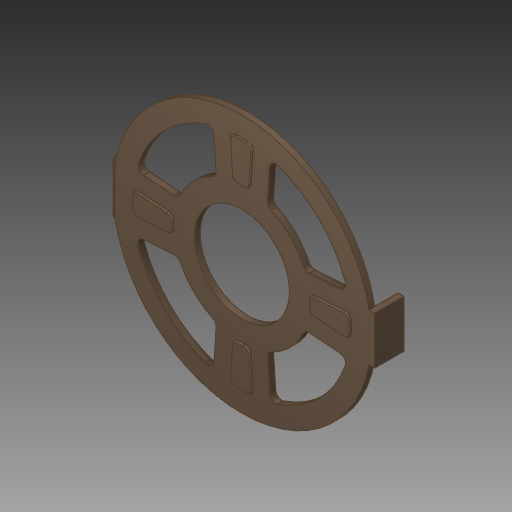
# Autodesk Inventor part: SŁONECZKO
Saved by Autodesk Inventor 2017 SP1 (Build 210196100, 196)
## iProperties
Created: 2021-01-06
Part Number: SŁONECZKO
Material: Stal
Document SubType Name: Modeling
Designer: Napoleon
Mass: 0.893655 g
Surface Area: 6.07713 cm^2
Volume: 0.113841 cm^3
Density: 7.85 g/cm^3
Appearance: Anodowany - brązowy
Author: Napoleon
Autodesk Inventor part; units mm, degrees
ref_plane "YZ Plane" through (0, 0, 0) normal (1, 0, 0) x (0, 1, 0)
ref_plane "XZ Plane" through (0, 0, 0) normal (0, 1, 0) x (-1, 0, 0)
ref_plane "XY Plane" through (0, 0, 0) normal (0, 0, 1) x (1, 0, 0)
sketch "Szkic1" plane through (0, 0, 0) normal (0, 0, 1) x (1, 0, 0)
  circle A0 centre (0, 0) radius 4.05
  line L0 (-11.3, 2.025) -> (-11.3, -2.025)
  line L1 (-10.8, 2.025) -> (-11.3, 2.025)
  line L2 (-9.2716, 0.9962) -> (-5.7517, 0.7466)
  line L3 (-9.0036, 2.4272) -> (-5.3787, 2.1701)
  line L4 (-9.2716, 0.9962) -> (-5.8, 0.75)
  line L5 (-9.2716, -0.9962) -> (-5.7517, -0.7466)
  line L6 (-9.0036, -2.4272) -> (-5.3787, -2.1701)
  line L7 (-9.2716, -0.9962) -> (-5.8, -0.75)
  line L8 (-2.4272, -9.0036) -> (-2.1701, -5.3787)
  line L9 (-0.9962, -9.2716) -> (-0.7466, -5.7517)
  line L10 (-0.9962, -9.2716) -> (-0.75, -5.8)
  line L11 (0.9962, -9.2716) -> (0.7466, -5.7517)
  line L12 (0.9962, -9.2716) -> (0.75, -5.8)
  line L13 (2.4272, -9.0036) -> (2.1701, -5.3787)
  line L14 (9.0036, -2.4272) -> (5.3787, -2.1701)
  line L15 (9.2716, -0.9962) -> (5.7517, -0.7466)
  line L16 (9.2716, -0.9962) -> (5.8, -0.75)
  line L17 (9.2716, 0.9962) -> (5.7517, 0.7466)
  line L18 (9.2716, 0.9962) -> (5.8, 0.75)
  line L19 (9.0036, 2.4272) -> (5.3787, 2.1701)
  line L20 (2.4272, 9.0036) -> (2.1701, 5.3787)
  line L21 (0.9962, 9.2716) -> (0.7466, 5.7517)
  line L22 (0.9962, 9.2716) -> (0.75, 5.8)
  line L23 (-0.9962, 9.2716) -> (-0.7466, 5.7517)
  line L24 (-0.9962, 9.2716) -> (-0.75, 5.8)
  line L25 (-2.4272, 9.0036) -> (-2.1701, 5.3787)
  arc A1 (0.9962, 9.2716) -> (-0.9962, 9.2716) centre (0, 0) ccw
  arc A2 (0.7466, 5.7517) -> (-0.7466, 5.7517) centre (0, 0) ccw
  arc A3 (5.3787, 2.1701) -> (2.1701, 5.3787) centre (0, 0) ccw
  arc A4 (9.0036, 2.4272) -> (2.4272, 9.0036) centre (0, 0) ccw
  arc A5 (9.2716, -0.9962) -> (9.2716, 0.9962) centre (0, 0) ccw
  arc A6 (5.7517, -0.7466) -> (5.7517, 0.7466) centre (0, 0) ccw
  arc A7 (2.4272, -9.0036) -> (9.0036, -2.4272) centre (0, 0) ccw
  arc A8 (2.1701, -5.3787) -> (5.3787, -2.1701) centre (0, 0) ccw
  arc A9 (-0.7466, -5.7517) -> (0.7466, -5.7517) centre (0, 0) ccw
  arc A10 (-0.9962, -9.2716) -> (0.9962, -9.2716) centre (0, 0) ccw
  arc A11 (-9.0036, -2.4272) -> (-2.4272, -9.0036) centre (0, 0) ccw
  arc A12 (-5.3787, -2.1701) -> (-2.1701, -5.3787) centre (0, 0) ccw
  arc A13 (-2.1701, 5.3787) -> (-5.3787, 2.1701) centre (0, 0) ccw
  arc A14 (-5.7517, 0.7466) -> (-5.7517, -0.7466) centre (0, 0) ccw
  arc A15 (-2.4272, 9.0036) -> (-9.0036, 2.4272) centre (0, 0) ccw
  arc A16 (-9.2716, 0.9962) -> (-9.2716, -0.9962) centre (0, 0) ccw
  line L26 (-10.8, -2.025) -> (-11.3, -2.025)
  arc A17 (-10.7083, -2.5164) -> (-2.5164, -10.7083) centre (0, 0) ccw
  arc A18 (-10.812, -2.025) -> (10.812, -2.025) centre (0, 0) ccw
  arc A19 (-2.5164, 10.7083) -> (-10.7083, 2.5164) centre (0, 0) ccw
  arc A20 (10.812, 2.025) -> (-10.812, 2.025) centre (0, 0) ccw
  line L27 (11.3, 2.025) -> (11.3, -2.025)
  line L28 (10.8, 2.025) -> (11.3, 2.025)
  line L29 (10.8, -2.025) -> (11.3, -2.025)
  dimension "d19" = 360
  constraints: 60 end point, 42 point on circle, 21 centre point, 4 point on line, 3 coincident, 65 other
extrude "Wyciągnięcie proste1" add sketch "Szkic1" against normal blind 0.5
fillet "Zaokrąglenie1" radius 0.5 32 edges at (-9.2716, 0.9962, -0.25) (-5.7517, 0.7466, -0.25) (-5.7517, -0.7466, -0.25) (-9.2716, -0.9962, -0.25) (-9.0036, 2.4272, -0.25) (-5.3787, 2.1701, -0.25) (-2.1701, 5.3787, -0.25) (-2.4272, 9.0036, -0.25) (-0.9962, 9.2716, -0.25) (-0.7466, 5.7517, -0.25) (0.7466, 5.7517, -0.25) (0.9962, 9.2716, -0.25) (2.4272, 9.0036, -0.25) (2.1701, 5.3787, -0.25) (5.3787, 2.1701, -0.25) (9.0036, 2.4272, -0.25) (5.7517, 0.7466, -0.25) (5.7517, -0.7466, -0.25) (9.2716, -0.9962, -0.25) (9.2716, 0.9962, -0.25) (5.3787, -2.1701, -0.25) (9.0036, -2.4272, -0.25) (2.1701, -5.3787, -0.25) (2.4272, -9.0036, -0.25) (-0.7466, -5.7517, -0.25) (0.7466, -5.7517, -0.25) (0.9962, -9.2716, -0.25) (-0.9962, -9.2716, -0.25) (-2.1701, -5.3787, -0.25) (-2.4272, -9.0036, -0.25) (-9.0036, -2.4272, -0.25) (-5.3787, -2.1701, -0.25)
sketch "Szkic2" plane through (0, 0, -0.5) normal (0, 0, -1) x (-1, 0, 0)
  line L0 (-11.3, 2.025) -> (-10.8, 2.025)
  line L1 (-11.3, 2.025) -> (-10.8, 2.025)
  line L2 (-10.8, 2.025) -> (-10.8, -2.025)
  line L3 (-10.8, -2.025) -> (-11.3, -2.025)
  line L4 (-11.3, -2.025) -> (-11.3, 2.025)
  line L5 (11.3, 2.025) -> (10.8, 2.025)
  line L6 (10.8, 2.025) -> (10.8, -2.025)
  line L7 (10.8, -2.025) -> (11.3, -2.025)
  line L8 (11.3, -2.025) -> (11.3, 2.025)
  circle A0 centre (0, 0) radius 4.05 projected
  arc A1 (-3.0447, 8.8139) -> (-8.8139, 3.0447) centre (0, 0) ccw projected
  arc A2 (-2.3827, 8.3767) -> (-3.0447, 8.8139) centre (-2.8815, 8.3413) ccw projected
  line L9 (-2.3827, 8.3767) -> (-2.1951, 5.7304) projected
  arc A3 (-2.48, 5.243) -> (-2.1951, 5.7304) centre (-2.6938, 5.695) ccw projected
  arc A4 (-2.48, 5.243) -> (-5.243, 2.48) centre (0, 0) ccw projected
  arc A5 (-5.7304, 2.1951) -> (-5.243, 2.48) centre (-5.695, 2.6938) ccw projected
  line L10 (-5.7304, 2.1951) -> (-8.3767, 2.3827) projected
  arc A6 (-8.8139, 3.0447) -> (-8.3767, 2.3827) centre (-8.3413, 2.8815) ccw projected
  arc A7 (-8.8139, -3.0447) -> (-3.0447, -8.8139) centre (0, 0) ccw projected
  arc A8 (-8.3767, -2.3827) -> (-8.8139, -3.0447) centre (-8.3413, -2.8815) ccw projected
  line L11 (-8.3767, -2.3827) -> (-5.7304, -2.1951) projected
  arc A9 (-5.243, -2.48) -> (-5.7304, -2.1951) centre (-5.695, -2.6938) ccw projected
  arc A10 (-5.243, -2.48) -> (-2.48, -5.243) centre (0, 0) ccw projected
  arc A11 (-2.1951, -5.7304) -> (-2.48, -5.243) centre (-2.6938, -5.695) ccw projected
  line L12 (-2.1951, -5.7304) -> (-2.3827, -8.3767) projected
  arc A12 (-3.0447, -8.8139) -> (-2.3827, -8.3767) centre (-2.8815, -8.3413) ccw projected
  arc A13 (3.0447, -8.8139) -> (8.8139, -3.0447) centre (0, 0) ccw projected
  arc A14 (2.3827, -8.3767) -> (3.0447, -8.8139) centre (2.8815, -8.3413) ccw projected
  line L13 (2.3827, -8.3767) -> (2.1951, -5.7304) projected
  arc A15 (2.48, -5.243) -> (2.1951, -5.7304) centre (2.6938, -5.695) ccw projected
  arc A16 (2.48, -5.243) -> (5.243, -2.48) centre (0, 0) ccw projected
  arc A17 (5.7304, -2.1951) -> (5.243, -2.48) centre (5.695, -2.6938) ccw projected
  line L14 (5.7304, -2.1951) -> (8.3767, -2.3827) projected
  arc A18 (8.8139, -3.0447) -> (8.3767, -2.3827) centre (8.3413, -2.8815) ccw projected
  arc A19 (5.243, 2.48) -> (2.48, 5.243) centre (0, 0) ccw projected
  arc A20 (2.1951, 5.7304) -> (2.48, 5.243) centre (2.6938, 5.695) ccw projected
  line L15 (2.1951, 5.7304) -> (2.3827, 8.3767) projected
  arc A21 (3.0447, 8.8139) -> (2.3827, 8.3767) centre (2.8815, 8.3413) ccw projected
  arc A22 (8.8139, 3.0447) -> (3.0447, 8.8139) centre (0, 0) ccw projected
  arc A23 (8.3767, 2.3827) -> (8.8139, 3.0447) centre (8.3413, 2.8815) ccw projected
  line L16 (8.3767, 2.3827) -> (5.7304, 2.1951) projected
  arc A24 (5.243, 2.48) -> (5.7304, 2.1951) centre (5.695, 2.6938) ccw projected
  arc A25 (0.4886, 9.3122) -> (-0.4886, 9.3122) centre (0, 0) ccw projected
  arc A26 (0.9612, 8.7775) -> (0.4886, 9.3122) centre (0.4624, 8.8129) ccw projected
  line L17 (0.9612, 8.7775) -> (0.7825, 6.2582) projected
  arc A27 (0.2612, 5.7941) -> (0.7825, 6.2582) centre (0.2838, 6.2936) ccw projected
  arc A28 (0.2612, 5.7941) -> (-0.2612, 5.7941) centre (0, 0) ccw projected
  arc A29 (-0.7825, 6.2582) -> (-0.2612, 5.7941) centre (-0.2838, 6.2936) ccw projected
  line L18 (-0.7825, 6.2582) -> (-0.9612, 8.7775) projected
  arc A30 (-0.4886, 9.3122) -> (-0.9612, 8.7775) centre (-0.4624, 8.8129) ccw projected
  arc A31 (-9.3122, 0.4886) -> (-9.3122, -0.4886) centre (0, 0) ccw projected
  arc A32 (-8.7775, 0.9612) -> (-9.3122, 0.4886) centre (-8.8129, 0.4624) ccw projected
  line L19 (-8.7775, 0.9612) -> (-6.2582, 0.7825) projected
  arc A33 (-5.7941, 0.2612) -> (-6.2582, 0.7825) centre (-6.2936, 0.2838) ccw projected
  arc A34 (-5.7941, 0.2612) -> (-5.7941, -0.2612) centre (0, 0) ccw projected
  arc A35 (-6.2582, -0.7825) -> (-5.7941, -0.2612) centre (-6.2936, -0.2838) ccw projected
  line L20 (-6.2582, -0.7825) -> (-8.7775, -0.9612) projected
  arc A36 (-9.3122, -0.4886) -> (-8.7775, -0.9612) centre (-8.8129, -0.4624) ccw projected
  arc A37 (-0.4886, -9.3122) -> (0.4886, -9.3122) centre (0, 0) ccw projected
  arc A38 (-0.9612, -8.7775) -> (-0.4886, -9.3122) centre (-0.4624, -8.8129) ccw projected
  line L21 (-0.9612, -8.7775) -> (-0.7825, -6.2582) projected
  arc A39 (-0.2612, -5.7941) -> (-0.7825, -6.2582) centre (-0.2838, -6.2936) ccw projected
  arc A40 (-0.2612, -5.7941) -> (0.2612, -5.7941) centre (0, 0) ccw projected
  arc A41 (0.7825, -6.2582) -> (0.2612, -5.7941) centre (0.2838, -6.2936) ccw projected
  line L22 (0.7825, -6.2582) -> (0.9612, -8.7775) projected
  arc A42 (0.4886, -9.3122) -> (0.9612, -8.7775) centre (0.4624, -8.8129) ccw projected
  arc A43 (9.3122, -0.4886) -> (9.3122, 0.4886) centre (0, 0) ccw projected
  arc A44 (8.7775, -0.9612) -> (9.3122, -0.4886) centre (8.8129, -0.4624) ccw projected
  line L23 (8.7775, -0.9612) -> (6.2582, -0.7825) projected
  arc A45 (5.7941, -0.2612) -> (6.2582, -0.7825) centre (6.2936, -0.2838) ccw projected
  arc A46 (5.7941, -0.2612) -> (5.7941, 0.2612) centre (0, 0) ccw projected
  arc A47 (6.2582, 0.7825) -> (5.7941, 0.2612) centre (6.2936, 0.2838) ccw projected
  line L24 (6.2582, 0.7825) -> (8.7775, 0.9612) projected
  arc A48 (9.3122, 0.4886) -> (8.7775, 0.9612) centre (8.8129, 0.4624) ccw projected
  line L25 (11.3, -2.025) -> (11.3, 2.025) projected
  line L26 (11.3, 2.025) -> (10.812, 2.025) projected
  arc A49 (10.812, 2.025) -> (-10.812, 2.025) centre (0, 0) ccw projected
  line L27 (-10.812, 2.025) -> (-11.3, 2.025) projected
  line L28 (-11.3, 2.025) -> (-11.3, -2.025) projected
  line L29 (-11.3, -2.025) -> (-10.812, -2.025) projected
  arc A50 (-10.812, -2.025) -> (10.812, -2.025) centre (0, 0) ccw projected
  line L30 (10.812, -2.025) -> (11.3, -2.025) projected
  constraints: 18 end point, 4 parallel, 2 horizontal, 2 perpendicular
extrude "Wyciągnięcie proste3" add sketch "Szkic2" along normal blind 2 contours L0 L2 L3 L4 | L5 L8 L7 L6
fillet "Zaokrąglenie4" radius 0.5 1 edges at (-11.3, 0, 0)
fillet "Zaokrąglenie6" radius 0.25 2 edges at (10.8, 0, -0.5) (-10.8, 0, -0.5)
sketch "Szkic3" plane through (0, 0, 0) normal (0, 0, 1) x (1, 0, 0)
  arc A0 (0.4886, 9.3122) -> (-0.4886, 9.3122) centre (0, 0) ccw projected
  arc A1 (0.9612, 8.7775) -> (0.4886, 9.3122) centre (0.4624, 8.8129) ccw projected
  line L0 (0.9612, 8.7775) -> (0.7825, 6.2582) projected
  arc A2 (0.2612, 5.7941) -> (0.7825, 6.2582) centre (0.2838, 6.2936) ccw projected
  arc A3 (0.2612, 5.7941) -> (-0.2612, 5.7941) centre (0, 0) ccw projected
  arc A4 (-0.7825, 6.2582) -> (-0.2612, 5.7941) centre (-0.2838, 6.2936) ccw projected
  line L1 (-0.7825, 6.2582) -> (-0.9612, 8.7775) projected
  arc A5 (-0.4886, 9.3122) -> (-0.9612, 8.7775) centre (-0.4624, 8.8129) ccw projected
  arc A6 (9.3122, -0.4886) -> (9.3122, 0.4886) centre (0, 0) ccw projected
  arc A7 (8.7775, -0.9612) -> (9.3122, -0.4886) centre (8.8129, -0.4624) ccw projected
  line L2 (8.7775, -0.9612) -> (6.2582, -0.7825) projected
  arc A8 (5.7941, -0.2612) -> (6.2582, -0.7825) centre (6.2936, -0.2838) ccw projected
  arc A9 (5.7941, -0.2612) -> (5.7941, 0.2612) centre (0, 0) ccw projected
  arc A10 (6.2582, 0.7825) -> (5.7941, 0.2612) centre (6.2936, 0.2838) ccw projected
  line L3 (6.2582, 0.7825) -> (8.7775, 0.9612) projected
  arc A11 (9.3122, 0.4886) -> (8.7775, 0.9612) centre (8.8129, 0.4624) ccw projected
  arc A12 (-0.4886, -9.3122) -> (0.4886, -9.3122) centre (0, 0) ccw projected
  arc A13 (-0.9612, -8.7775) -> (-0.4886, -9.3122) centre (-0.4624, -8.8129) ccw projected
  line L4 (-0.9612, -8.7775) -> (-0.7825, -6.2582) projected
  arc A14 (-0.2612, -5.7941) -> (-0.7825, -6.2582) centre (-0.2838, -6.2936) ccw projected
  arc A15 (-0.2612, -5.7941) -> (0.2612, -5.7941) centre (0, 0) ccw projected
  arc A16 (0.7825, -6.2582) -> (0.2612, -5.7941) centre (0.2838, -6.2936) ccw projected
  line L5 (0.7825, -6.2582) -> (0.9612, -8.7775) projected
  arc A17 (0.4886, -9.3122) -> (0.9612, -8.7775) centre (0.4624, -8.8129) ccw projected
  arc A18 (-9.3122, 0.4886) -> (-9.3122, -0.4886) centre (0, 0) ccw projected
  arc A19 (-8.7775, 0.9612) -> (-9.3122, 0.4886) centre (-8.8129, 0.4624) ccw projected
  line L6 (-8.7775, 0.9612) -> (-6.2582, 0.7825) projected
  arc A20 (-5.7941, 0.2612) -> (-6.2582, 0.7825) centre (-6.2936, 0.2838) ccw projected
  arc A21 (-5.7941, 0.2612) -> (-5.7941, -0.2612) centre (0, 0) ccw projected
  arc A22 (-6.2582, -0.7825) -> (-5.7941, -0.2612) centre (-6.2936, -0.2838) ccw projected
  line L7 (-6.2582, -0.7825) -> (-8.7775, -0.9612) projected
  arc A23 (-9.3122, -0.4886) -> (-8.7775, -0.9612) centre (-8.8129, -0.4624) ccw projected
extrude "Wyciągnięcie proste4" add sketch "Szkic3" along normal blind 0.1
fillet "Zaokrąglenie7" radius 0.099 32 edges at (-0.6162, 5.9202, 0.1) (0, 5.8, 0.1) (0.6162, 5.9202, 0.1) (0.8718, 7.5179, 0.1) (0.8371, 9.144, 0.1) (0, 9.325, 0.1) (-0.8371, 9.144, 0.1) (-0.8718, 7.5179, 0.1) (-0.8371, -9.144, 0.1) (-0.8718, -7.5179, 0.1) (-0.6162, -5.9202, 0.1) (0, -5.8, 0.1) (0.6162, -5.9202, 0.1) (0.8718, -7.5179, 0.1) (0.8371, -9.144, 0.1) (0, -9.325, 0.1) (9.144, -0.8371, 0.1) (7.5179, -0.8718, 0.1) (5.9202, -0.6162, 0.1) (5.8, 0, 0.1) (5.9202, 0.6162, 0.1) (7.5179, 0.8718, 0.1) (9.144, 0.8371, 0.1) (9.325, 0, 0.1) (-9.144, 0.8371, 0.1) (-7.5179, 0.8718, 0.1) (-5.9202, 0.6162, 0.1) (-5.8, 0, 0.1) (-5.9202, -0.6162, 0.1) (-7.5179, -0.8718, 0.1) (-9.144, -0.8371, 0.1) (-9.325, 0, 0.1)
